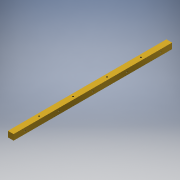
# Autodesk Inventor part: mounting rail 7.0 x.250 x .250_092717
Saved by Autodesk Inventor 2017 (Build 210142000, 142)
## iProperties
Created: 2014-01-27
Part Number: mounting rail 7.0 x.250 x .250_092717
Material: Gold
Document SubType Name: Modeling
Designer: rtreacy
Density: 1 g/cm^3
Appearance: Gold - Metal
Author: rtreacy
Autodesk Inventor part; units mm, degrees
ref_plane "YZ Plane" through (0, 0, 0) normal (1, 0, 0) x (0, 1, 0)
ref_plane "XZ Plane" through (0, 0, 0) normal (0, 1, 0) x (-1, 0, 0)
ref_plane "XY Plane" through (0, 0, 0) normal (0, 0, 1) x (1, 0, 0)
sketch "Sketch1" plane through (0, 0, 0) normal (0, 0, 1) x (1, 0, 0)
  line L0 (-7.6953, 6.4307) -> (-1.3453, 6.4307)
  line L1 (-1.3453, 6.4307) -> (-1.3453, 0.0807)
  line L2 (-1.3453, 0.0807) -> (-7.6953, 0.0807)
  line L3 (-7.6953, 0.0807) -> (-7.6953, 6.4307)
  point P0 (0, 0)
  dimension "d0" = 6.35
  dimension "d2" = 6.35
  constraints: 8 end point, 2 parallel, 1 horizontal, 1 perpendicular
  measures "d0" distance of L0.start L0.end
  measures "d2" distance of L2.end L0.start
extrude "Extrusion1" add sketch "Sketch1" along normal blind 177.8
sketch "Sketch2" plane through (-1.3453, 0.0807, 0) normal (1, 0, 0) x (0, 0, -1)
  point P0 (-177.8, 6.35)
  point P1 (0, -0.0807)
  point P2 (-165.1, 3.175)
  dimension "d5" = 3.175
  dimension "d6" = 12.7
  measures "d5" vertical distance of point (-177.8, 6.35) point (-165.1, 3.175)
  measures "d6" horizontal distance of point (-165.1, 3.175) point (-177.8, 6.35)
hole "Hole1" at (-1.3453, 3.2557, 165.1) direction (-1, 0, 0) diameter 1.7018 end through all
pattern_linear "Rectangular Pattern1" count 5 spacing 38.1 along (0, 0, -1) of "Hole1"
sketch "Sketch3" plane through (160.5797, 6.4307, 92.075) normal (0, 1, 0) x (1, 0, 0)
  point P0 (0, -0.0807)
  point P1 (-165.1, -53.975)
  point P2 (-161.925, -85.725)
  point P3 (-168.275, -85.725)
  dimension "d33" = 31.75
  dimension "d37" = 3.175
  measures "d33" vertical distance of point (-161.925, -85.725) point (-165.1, -53.975)
  measures "d37" horizontal distance of point (-168.275, -85.725) point (-165.1, -53.975)
hole "Hole2" at (-4.5203, 6.4307, 146.05) direction (0, -1, 0) diameter 1.7018 end through all
pattern_linear "Rectangular Pattern2" count 4 spacing 38.1 along (0, 0, -1) of "Hole2"
body "Solid1"
